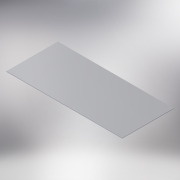
# Autodesk Inventor part: baseplate-alu
Saved by Autodesk Inventor 2016 (Build 200138000, 138)
## iProperties
Created: 2015-05-03
Part Number: baseplate-alu
Material: Aluminum 6061
Document SubType Name: Modeling
Designer: ax
Mass: 2916 g
Surface Area: 7278 cm^2
Volume: 1080 cm^3
Density: 2.7 g/cm^3
Appearance: Aluminum - Flat
Author: ax
Autodesk Inventor part; units mm, degrees
ref_plane "YZ Plane" through (0, 0, 0) normal (1, 0, 0) x (0, 1, 0)
ref_plane "XZ Plane" through (0, 0, 0) normal (0, 1, 0) x (-1, 0, 0)
ref_plane "XY Plane" through (0, 0, 0) normal (0, 0, 1) x (1, 0, 0)
sketch "Sketch1" plane through (0, 0, 0) normal (0, 0, 1) x (1, 0, 0)
  line L0 (0, 0) -> (900, 0)
  line L1 (900, 0) -> (900, 400)
  line L2 (900, 400) -> (0, 400)
  line L3 (0, 400) -> (0, 0)
  dimension "d0" = 900
  dimension "d1" = 400
  constraints: 8 end point, 2 parallel, 1 horizontal, 1 perpendicular
  measures "d0" distance of L2.end L1.end
  measures "d1" distance of L1.end L0.end
extrude "Extrusion1" add sketch "Sketch1" along normal blind 3
body "Solid1"
